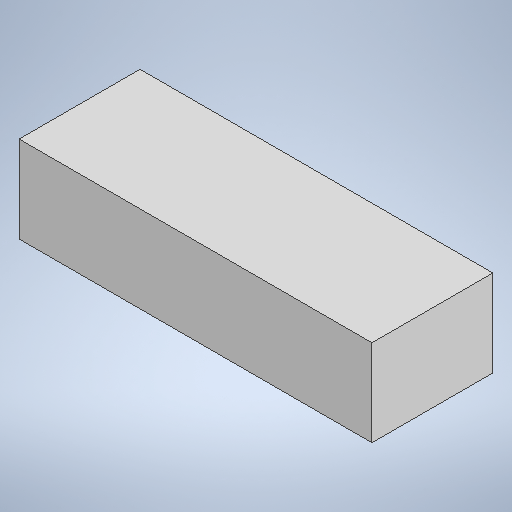
# Autodesk Inventor part: Battery for Water Sensor
Saved by Autodesk Inventor 2025 (Build 290162000, 162)
## iProperties
Created: 2024-07-10
Part Number: Battery for Water Sensor
Material: Generic
Document SubType Name: Modeling
Designer: track
Density: 1 g/cm^3
Appearance: Default
Author: track
Autodesk Inventor part; units mm, degrees
ref_plane "YZ Plane" through (0, 0, 0) normal (1, 0, 0) x (0, 1, 0)
ref_plane "XZ Plane" through (0, 0, 0) normal (0, 1, 0) x (-1, 0, 0)
ref_plane "XY Plane" through (0, 0, 0) normal (0, 0, 1) x (1, 0, 0)
sketch "Sketch1" plane through (0, 0, 0) normal (0, 1, 0) x (-1, 0, 0)
  line L0 (-54, -18.5) -> (54, -18.5)
  line L1 (54, -18.5) -> (54, 18.5)
  line L2 (54, 18.5) -> (-54, 18.5)
  line L3 (-54, 18.5) -> (-54, -18.5)
  line L4 (-54, -18.5) -> (54, 18.5) construction
  line L5 (54, -18.5) -> (-54, 18.5) construction
  point P0 (0, 0)
  dimension "d0" = 108
  dimension "d1" = 37
  constraints: 12 end point, 2 midpoint, 2 parallel, 1 horizontal, 1 perpendicular
  measures "d0" distance of L1.end L2.end
  measures "d1" distance of L2.end L0.start
extrude "Extrusion1" add sketch "Sketch1" along normal blind 26.5
body "Solid1"
